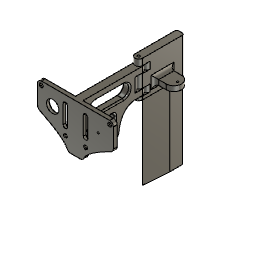
rudder (Autodesk Fusion 360 design; units mm, degrees)
Autodesk Fusion 360 part; units mm, degrees
sketch "Sketch1" plane through (0, 0, 0) normal (0, 0, 1) x (1, 0, 0)
  line L0 (0, 0) -> (60, 0)
  line L1 (60, 0) -> (60, 3)
  line L2 (0, 3) -> (0, 0)
  line L3 (30, 3) -> (30, 53) construction
  line L4 (30, 53) -> (33, 53) construction
  line L5 (30, 53) -> (27, 53) construction
  line L6 (27, 53) -> (33, 53)
  line L7 (33, 53) -> (33, 3)
  line L8 (27, 53) -> (27, 3)
  line L9 (60, 3) -> (33, 3)
  line L10 (27, 3) -> (0, 3)
  dimension "d1" = 60
  dimension "d2" = 3
  dimension "d3" = 50
  dimension "d4" = 3
  dimension "d5" = 3
  constraint horizontal L0
  constraint vertical L1
  constraint horizontal L9
  constraint vertical L2
  constraint coincident L0.start L2.end
  constraint perpendicular L3 L9
  constraint perpendicular L3 L4
  constraint perpendicular L3 L5
  constraint perpendicular L7 L9
  constraint coincident L8.end L9
  constraint perpendicular L8 L9
  constraint collinear L9 L10
  measures "d1" distance of L0.start L0.end
  measures "d2" distance of L0.start L2.start
  measures "d3" distance of L3.start L3.end
  measures "d4" distance of L3.end L4.end
  measures "d5" distance of L3.end L5.end
extrude "Extrude1" add sketch "Sketch1" along normal blind 20 makes body 1
sketch "Sketch2" plane through (33, 0, 0) normal (1, 0, 0) x (0, 1, 0)
  line L0 (3, 0) -> (53, 0)
  line L1 (53, 0) -> (53, 20)
  line L2 (53, 20) -> (3, 20)
  line L3 (3, 20) -> (3, 0)
  line L4 (53, 20) -> (53, 15.5) construction
  line L5 (53, 0) -> (53, 4.5) construction
  line L6 (53, 4.5) -> (47, 4.5)
  line L7 (47, 4.5) -> (47, 15.5)
  line L8 (47, 15.5) -> (53, 15.5)
  line L9 (53, 15.5) -> (53, 4.5)
  dimension "d8" = 4.5
  dimension "d9" = 4.5
  dimension "d10" = 6
  constraint coincident L1.end L2.start
  constraint perpendicular L2 L4
  constraint coincident L0.end L1.start
  constraint perpendicular L2 L5
  constraint horizontal L6
  constraint vertical L7
  constraint horizontal L8
  constraint vertical L9
  measures "d8" distance of L1.end L4.end
  measures "d9" distance of L0.end L5.end
  measures "d10" distance of L5.end L6.end
extrude "Extrude2" cut sketch "Sketch2" against normal blind 6 contours L1 L6 L7 L8 L9 bodies 1
fillet "Fillet2" radius 3 4 edges at (27, 53, 2.25) (27, 53, 17.75) (33, 53, 2.25) (33, 53, 17.75) on bodies 1
sketch "Sketch4" plane through (0, 0, 20) normal (0, 0, 1) x (-1, 0, 0)
  arc A0 (-33, -50) -> (-27, -50) centre (-30, -50) ccw
  line L0 (-27, -50) -> (-27, -3)
  line L1 (-27, -3) -> (0, -3)
  line L2 (0, 0) -> (-60, 0)
  line L3 (-60, -3) -> (-33, -3)
  line L4 (-33, -3) -> (-33, -50)
  circle A1 centre (-30, -50) radius 1.25
  line L5 (0, -3) -> (0, 0)
  line L6 (-60, 0) -> (-60, -3)
  dimension "d17" = 2.5
  constraint concentric A0 A1
  measures "d17" diameter of A1
extrude "Extrude3" cut sketch "Sketch4" against normal blind 20 contours A1 bodies 1
sketch "Sketch10" plane through (0, 3, 0) normal (0, 1, 0) x (-1, 0, 0)
  line L0 (-27, 0) -> (0, 0)
  line L1 (0, 0) -> (0, 20)
  line L2 (0, 20) -> (-27, 20)
  line L3 (-27, 20) -> (-27, 0)
sketch "Sketch11" plane through (0, 3, 0) normal (0, 1, 0) x (-1, 0, 0)
  line L0 (-33, 20) -> (-60, 20)
  line L1 (-60, 20) -> (-60, 0)
  line L2 (-60, 0) -> (-33, 0)
  line L3 (-33, 0) -> (-33, 20)
sketch "Sketch14" plane through (0, 0, 0) normal (1, 0, 0) x (0, 1, 0)
  line L0 (90.0644, 25) -> (120.0644, 25)
  line L1 (120.0644, 25) -> (120.0644, -65)
  line L2 (120.0644, -65) -> (90.0644, -65)
  line L3 (90.0644, 25) -> (84.0644, 25)
  line L4 (84.0644, -3.5) -> (90.0644, -3.5)
  line L5 (84.0644, 25) -> (84.0644, 20) construction
  line L6 (84.0644, -3.5) -> (84.0644, -1) construction
  line L7 (84.0644, 20) -> (84.0644, 14.5) construction
  line L8 (84.0644, 4.5) -> (90.0644, 4.4065)
  line L9 (84.0644, 14.5) -> (90.0644, 14.5)
  line L10 (84.0644, -1) -> (90.0644, -1)
  line L11 (84.0644, 20) -> (90.0645, 20)
  line L12 (84.0644, 25) -> (84.0644, 20)
  line L13 (84.0644, 14.5) -> (84.0644, 4.5)
  line L14 (84.0644, -1) -> (84.0644, -3.5)
  line L15 (90.0644, -1) -> (90.0644, 4.4065)
  line L16 (90.0644, 14.5) -> (90.0644, 20)
  line L17 (90.0644, 14.5) -> (90.0644, 20)
  line L18 (90.0644, -65) -> (90.0644, -3.5)
  line L19 (90.0644, -1) -> (90.0644, 4.4065)
  line L20 (90.0644, -3.5) -> (120.0644, -3.5)
  dimension "d43" = 30
  dimension "d44" = 90
  dimension "d45" = 6
  dimension "d46" = 28.5
  dimension "d47" = 2.5
  dimension "d48" = 5.5
  dimension "d49" = 5.5
  dimension "d50" = 6
  constraint horizontal L0
  constraint vertical L1
  constraint horizontal L2
  constraint vertical L18
  constraint horizontal L3
  constraint vertical L12
  constraint horizontal L4
  constraint vertical L15
  constraint perpendicular L4 L6
  constraint perpendicular L3 L7
  constraint horizontal L9
  constraint horizontal L10
  constraint horizontal L11
  constraint collinear L12 L13
  constraint collinear L13 L14
  constraint collinear L15 L16
  constraint collinear L17 L18
  constraint coincident L11 L16.end
  constraint coincident L10 L15.start
  constraint collinear L18 L19
  constraint coincident L1 L20.end
  constraint perpendicular L1 L20
  measures "d43" distance of L0.start L0.end
  measures "d44" distance of L0.start L2.end
  measures "d45" distance of L0.start L3.end
  measures "d46" distance of L0.start L4.end
  measures "d47" distance of L4.start L6.end
  measures "d48" distance of L6.end L8.start
  measures "d49" distance of L5.end L7.end
  measures "d50" distance of L7.end L9.end
extrude "Extrude9" add sketch "Sketch14" along normal mid plane 6 separate body contours L0 L1 L3 L4 L8 L9 L10 L11 L12 L13 L14 L15 L16 L17 L19 L20 makes body 2
extrude "Extrude10" add sketch "Sketch14" along normal mid plane 3 contours L1 L2 L18 L20 bodies 2
fillet "Fillet7" radius 3 6 edges at (-3, 84.0644, 22.5) (3, 84.0644, 22.5) (3, 84.0644, 9.5) (-3, 84.0644, 9.5) (-3, 84.0644, -2.25) (3, 84.0644, -2.25) on bodies 2
sketch "Sketch16" plane through (0, 0, 25) normal (0, 0, 1) x (-1, 0, 0)
  arc A0 (3, -87.0644) -> (-3, -87.0644) centre (0, -87.0644) ccw
  line L0 (-3, -87.0644) -> (-3, -120.0644)
  line L1 (-3, -120.0644) -> (3, -120.0644)
  line L2 (3, -120.0644) -> (3, -87.0644)
  circle A1 centre (0, -87.0644) radius 1
  dimension "d58" = 2
  constraint concentric A0 A1
  measures "d58" diameter of A1
extrude "Extrude11" cut sketch "Sketch16" against normal blind 31 contours A1 bodies 2
sketch "Sketch17" plane through (0, 0, -65) normal (0, 0, -1) x (1, 0, 0)
  line L0 (-1.5, -120.0644) -> (1.5, -120.0644)
  line L1 (1.5, -120.0644) -> (1.5, -90.0644)
  line L2 (1.5, -90.0644) -> (-1.5, -90.0644)
  line L3 (-1.5, -90.0644) -> (-1.5, -120.0644)
  line L4 (0, -90.0644) -> (0, -110.0644) construction
  line L5 (0, -110.0644) -> (1.5, -110.0644) construction
  line L6 (0, -110.0644) -> (-1.5, -110.0644) construction
  line L7 (30, 110) -> (30, 470) construction
  line L8 (0, -90.0644) -> (1.5, -110.0644)
  line L9 (0, -90.0644) -> (-1.5, -110.0644)
  dimension "d62" = 20
  constraint midpoint L2 L4.start
  constraint perpendicular L2 L4
  constraint coincident L1 L5.end
  constraint perpendicular L1 L5
  constraint coincident L3 L6.end
  constraint perpendicular L3 L6
  constraint perpendicular L6 L7
  measures "d62" distance of L4.start L4.end
extrude "Extrude12" cut sketch "Sketch17" against normal blind 61.5 contours L2 L3 L9 | L1 L2 L8 bodies 2
fillet "Fillet9" radius 1 4 edges at (0.75, 100.0644, -3.5) (1.5, 115.0644, -3.5) (-0.75, 100.0644, -3.5) (-1.5, 115.0644, -3.5) on bodies 2
fillet "Fillet10" radius 1.5 2 edges at (3, 120.0644, 10.75) (-3, 120.0644, 10.75) on bodies 2
sketch "Sketch19" plane through (3, 0, 0) normal (1, 0, 0) x (0, 1, 0)
  line L0 (118.5644, -3.5) -> (118.5644, 25)
  line L1 (118.5644, 25) -> (87.0644, 25)
  line L2 (87.0644, 25) -> (87.0644, 20)
  line L3 (87.0644, 20) -> (90.0644, 20)
  line L4 (90.0644, 20) -> (90.0644, 14.5)
  line L5 (90.0644, 14.5) -> (87.0644, 14.5)
  line L6 (87.0644, 14.5) -> (87.0644, 4.4532)
  line L7 (87.0644, 4.4532) -> (90.0644, 4.4065)
  line L8 (90.0644, 4.4065) -> (90.0644, -1)
  line L9 (90.0644, -1) -> (87.0644, -1)
  line L10 (87.0644, -1) -> (87.0644, -3.5)
  line L11 (87.0644, -3.5) -> (118.5644, -3.5)
  line L12 (87.0644, 9.4766) -> (118.5644, 10.75) construction
  line L13 (108.8144, 6.9899) -> (96.8144, 6.9899)
  line L14 (108.8144, 6.9899) -> (120, 6.9899) construction
  line L15 (108.8144, 6.9899) -> (96.8144, 6.9899)
  line L16 (96.8144, 6.9899) -> (96.8144, 2.9899)
  line L17 (96.8144, 2.9899) -> (108.8144, 2.9899)
  line L18 (108.8144, 2.9899) -> (108.8144, 6.9899)
  point P0 (102.8144, 10.1133)
  dimension "d122" = 12
  dimension "d123" = 4
  constraint midpoint L6 L12.start
  constraint midpoint L0 L12.end
  constraint horizontal L13
  constraint midpoint L12 P0
  constraint perpendicular L0 L14
  constraint horizontal L15
  constraint vertical L16
  constraint horizontal L17
  constraint vertical L18
  measures "d122" distance of L13.start L13.end
  measures "d123" distance of L13.start L17.end
extrude "Extrude14" add sketch "Sketch19" along normal blind 15 contours L13 L15 L16 L17 L18 bodies 2
fillet "Fillet14" radius 3 4 edges at (-3, 90.0644, 1.7032) (-3, 90.0644, 17.25) (3, 90.0644, 17.25) (3, 90.0644, 1.7032) on bodies 2
sketch "Sketch23" plane through (0, 0, 0) normal (0, -1, 0) x (1, 0, 0)
  line L0 (0, 20) -> (0, 0)
  line L1 (0, 0) -> (60, 0)
  line L2 (60, 0) -> (60, 20)
  line L3 (60, 20) -> (0, 20)
  line L4 (3, 17) -> (57, 17) construction
  line L5 (30, 17) -> (57, 17) construction
  line L6 (57, 17) -> (3, 17) construction
  line L7 (30, 20) -> (30, -30) construction
  circle A0 centre (3, 17) radius 1.5
  circle A1 centre (57, 17) radius 1.5
  line L8 (18, 0) -> (42, 0)
  line L9 (30, 17) -> (30, -8) construction
  line L10 (30, -8) -> (38, -8) construction
  line L11 (30, -8) -> (22, -8) construction
  circle A2 centre (38, -8) radius 1.5
  circle A3 centre (22, -8) radius 1.5
  line L12 (30, -18) -> (24, -18)
  line L13 (30, -18) -> (36, -18)
  spline S0 degree 5 poles (24, -18) (23.9428, -17.6951) (23.7865, -17.08) (23.4264, -16.1409) (22.6907, -14.8553) (21.3234, -13.1901) (19.4864, -11.4635) (17.1816, -9.6759) (14.4461, -7.8321) (11.3264, -5.9383) (7.8686, -4.0003) (4.8605, -2.4184) (2.4785, -1.2155) (0.8353, -0.4064) (0, 0) knots 0 0 0 0 0 0 0.1 0.2 0.3 0.4 0.5 0.6 0.7 0.8 0.9 1 1 1 1 1 1
  spline S1 degree 5 poles (36, -18) (36.0572, -17.6951) (36.2135, -17.08) (36.5736, -16.1409) (37.3093, -14.8553) (38.6766, -13.1901) (40.5136, -11.4635) (42.8184, -9.6759) (45.5539, -7.8321) (48.6736, -5.9383) (52.1314, -4.0003) (55.1395, -2.4184) (57.5215, -1.2155) (59.1647, -0.4064) (60, 0) knots 0 0 0 0 0 0 0.1 0.2 0.3 0.4 0.5 0.6 0.7 0.8 0.9 1 1 1 1 1 1
  line L14 (24.4672, -20.4896) -> (23.5328, -15.5104)
  line L15 (3.7531, -1.8254) -> (-3.7531, 1.8254)
  line L16 (35.5328, -20.4896) -> (36.4672, -15.5104)
  line L17 (56.2469, -1.8254) -> (63.7531, 1.8254)
  point P0 (18, 0)
  point P1 (42, 0)
  point P2 (30, -18)
  point P3 (20, -12)
  point P4 (40, -12)
  dimension "d89" = 3
  dimension "d90" = 3
  dimension "d93" = 12
  dimension "d94" = 12
  dimension "d171" = 25
  dimension "d172" = 8
  dimension "d173" = 8
  dimension "d174" = 3
  dimension "d175" = 3
  dimension "d176" = 20
  dimension "d179" = 38
  dimension "d180" = 6
  dimension "d181" = 6
  constraint midpoint L4 L5.start
  constraint midpoint L3 L7.start
  constraint perpendicular L1 L7
  constraint coincident L4.start L6.end
  constraint coincident L4.end L5.end
  constraint coincident L1 P0
  constraint coincident L1 P1
  constraint horizontal L8
  constraint coincident P0 L8.start
  constraint perpendicular L1 L9
  constraint perpendicular L9 L10
  constraint perpendicular L7 L11
  constraint coincident L10.end A2.centre
  constraint coincident L11.end A3.centre
  constraint coincident L7 P2
  constraint coincident P2 L12.start
  constraint perpendicular L7 L12
  constraint perpendicular L7 L13
  constraint coincident L0.end L1.start
  constraint midpoint L12.end L14
  constraint midpoint L0.end L15
  constraint symmetric L7 L12.end L13.end
  constraint symmetric L7 P3 P4
  constraint symmetric L7 L0.end L1.end
  constraint symmetric L7 L14.start L16.start
  constraint symmetric L7 L14.end L16.end
  constraint symmetric L7 L15.start L17.start
  constraint symmetric L7 L15.end L17.end
  measures "d89" diameter of A0
  measures "d90" diameter of A1
  measures "d93" distance of L7 P0
  measures "d94" distance of L7 P1
  measures "d171" distance of L5.start L9.end
  measures "d172" distance of L9.end L10.end
  measures "d173" distance of L9.end L11.end
  measures "d174" diameter of A2
  measures "d175" diameter of A3
  measures "d176" distance of L0.end L0.start
  measures "d179" distance of L7.start P2
  measures "d180" distance of P2 L12.end
  measures "d181" distance of P2 L13.end
extrude "Extrude17" add sketch "Sketch23" against normal blind 3 contours L0 L1 L2 L3 L8 | A0 | A1 bodies 1
extrude "Extrude18" cut sketch "Sketch23" against normal blind 3 contours A0 | A1 bodies 1
fillet "Fillet15" radius 3 2 edges at (33, 47, 10) (27, 47, 10) on bodies 1
sketch "Sketch24" plane through (0, 3, 0) normal (0, 1, 0) x (-1, 0, 0)
  circle A0 centre (-3, 17) radius 1.5
  circle A1 centre (-57, 17) radius 1.5
  line L0 (0, 20) -> (-27, 20)
  line L1 (-60, 20) -> (-60, 0)
  line L2 (0, 0) -> (0, 20)
  line L3 (-60, 0) -> (-33, 0)
  line L4 (-57, 17) -> (-48, 17) construction
  line L5 (-48, 17) -> (-48, 7) construction
  circle A2 centre (-48, 7) radius 2
  circle A3 centre (-48, 7) radius 0.75
  line L6 (-27, 20) -> (-27, 0)
  line L7 (-33, 0) -> (-33, 20)
  line L8 (-33, 20) -> (-60, 20)
  line L9 (-27, 0) -> (0, 0)
  point P0 (-30, 17)
  dimension "d101" = 9
  dimension "d102" = 10
  dimension "d103" = 4
  dimension "d109" = 18
  dimension "d116" = 1.5
  constraint coincident A1.centre L4.start
  constraint parallel L0 L4
  constraint perpendicular L4 L5
  constraint coincident L5.end A2.centre
  measures "d101" distance of A1.centre L4.end
  measures "d102" distance of L4.end L5.end
  measures "d103" diameter of A2
  measures "d109" distance of L4.end P0
  measures "d116" diameter of A3
ref_plane "WorkPlane1" through (3, 13, 17) normal (0, 1, 0) x (-1, 0, 0)
sketch "Sketch27" plane through (48, 13, 7) normal (0, 1, 0) x (1, 0, 0)
  circle A0 centre (0, 0) radius 1.5
  dimension "d115" = 3
  constraint coincident A0.centre origin
  measures "d115" diameter of A0
loft "Loft4" add profiles "Sketch24", "Sketch27" section 1 contours A2 | A3 section 2 bodies 1
extrude "Extrude21" cut sketch "Sketch24" along normal blind 12 and the other way blind 3 contours A3 bodies 1
fillet "Fillet16" radius 3 1 edges at (49.8647, 3, 7.7232) on bodies 1
sketch "Sketch28" plane through (0, 0, 6.9899) normal (0, 0, 1) x (-1, 0, 0)
  line L0 (-3, -108.8144) -> (-3, -96.8144)
  line L1 (-3, -96.8144) -> (-18, -96.8144)
  line L2 (-18, -96.8144) -> (-18, -108.8144)
  line L3 (-18, -108.8144) -> (-3, -108.8144)
  line L4 (-3, -102.8144) -> (-15, -102.8144) construction
  circle A0 centre (-15, -102.8144) radius 0.75
  dimension "d124" = 12
  dimension "d125" = 1.5
  constraint midpoint L0 L4.start
  constraint perpendicular L2 L4
  constraint coincident L4.end A0.centre
  measures "d124" distance of L4.start L4.end
  measures "d125" diameter of A0
extrude "Extrude22" cut sketch "Sketch28" against normal blind 4 contours A0 bodies 2
fillet "Fillet17" radius 6 2 edges at (18, 108.8144, 4.9899) (18, 96.8144, 4.9899) on bodies 2
fillet "Fillet18" radius 3 4 edges at (3, 102.8144, 6.9899) (3, 108.8144, 4.9899) (3, 102.8144, 2.9899) (3, 96.8144, 4.9899) on bodies 2
sketch "Sketch29" plane through (30, 3, 0) normal (0, 1, 0) x (-1, 0, 0)
  line L0 (0, -20.8667) -> (0, 0) construction
  circle A0 centre (-18, 7) radius 4.8537
  line L1 (0, 20) -> (0, -30)
  circle A1 centre (18, 7) radius 4.8537
  point P0 (0, -9.8667)
  point P1 (0, -3.8667)
  point P2 (0, -3.8667)
  point P3 (0, -9.8667)
  constraint coincident L0.end origin
  constraint vertical L0
  constraint coincident L0 P0
  constraint coincident L0 P2
  constraint coincident P2 P1
  constraint coincident P0 P3
  constraint symmetric A0 L1 A1
sketch "Sketch30" plane through (33, 0, 0) normal (1, 0, 0) x (0, 1, 0)
  line L0 (44, 15.5) -> (50, 15.5)
  line L1 (50, 15.5) -> (50, 20)
  line L2 (50, 20) -> (3, 20)
  line L3 (3, 20) -> (3, 0)
  line L4 (3, 0) -> (50, 0)
  line L5 (50, 0) -> (50, 4.5)
  line L6 (50, 4.5) -> (44, 4.5)
  line L7 (44, 4.5) -> (44, 15.5)
  line L8 (3, 20) -> (31, 20) construction
  line L9 (3, 20) -> (3, -18) construction
  line L10 (3, -18) -> (3, 0)
  line L11 (3, 0) -> (31, 0)
  line L12 (31, 0) -> (43, 0)
  line L13 (9, 0) -> (9, -18.4286) construction
  line L14 (17.5, 0) -> (17.5, -18.9835) construction
  line L15 (26, 0) -> (26, -19.5556) construction
  line L16 (6.5, -3.5) -> (6.5, -12.9286)
  arc A0 (6.5, -12.9286) -> (11.5, -12.9286) centre (9, -12.9286) ccw
  line L17 (11.5, -12.9286) -> (11.5, -3.5)
  arc A1 (11.5, -3.5) -> (6.5, -3.5) centre (9, -3.5) ccw
  line L18 (9, -1) -> (9, -15.4286) construction
  line L19 (15, -3.5) -> (15, -13.4835)
  arc A2 (15, -13.4835) -> (20, -13.4835) centre (17.5, -13.4835) ccw
  line L20 (20, -13.4835) -> (20, -3.5)
  arc A3 (20, -3.5) -> (15, -3.5) centre (17.5, -3.5) ccw
  line L21 (17.5, -1) -> (17.5, -15.9835) construction
  line L22 (23.5, -3.5) -> (23.5, -14.0556)
  arc A4 (23.5, -14.0556) -> (28.5, -14.0556) centre (26, -14.0556) ccw
  line L23 (28.5, -14.0556) -> (28.5, -3.5)
  arc A5 (28.5, -3.5) -> (23.5, -3.5) centre (26, -3.5) ccw
  line L24 (26, -1) -> (26, -16.5556) construction
  line L25 (44, 10) -> (3, 10) construction
  line L26 (13, 5) -> (35, 5)
  arc A6 (35, 5) -> (35, 15) centre (35, 10) ccw
  line L27 (35, 15) -> (13, 15)
  arc A7 (13, 15) -> (13, 5) centre (13, 10) ccw
  line L28 (8, 10) -> (40, 10) construction
  line L29 (31, 20) -> (31, -19) construction
  line L30 (3, -18) -> (31, -19)
  spline S0 degree 5 poles (31, -19) (31.0483, -18.3567) (31.1609, -17.0921) (31.3778, -15.261) (31.7645, -12.9536) (32.4223, -10.3089) (33.2722, -7.928) (34.3339, -5.8381) (35.6241, -4.062) (37.1446, -2.6021) (38.8825, -1.4409) (40.4347, -0.7344) (41.6846, -0.3222) (42.5553, -0.0988) (43, 0) knots 0 0 0 0 0 0 0.1 0.2 0.3 0.4 0.5 0.6 0.7 0.8 0.9 1 1 1 1 1 1
  point P0 (3, 20)
  point P1 (3, 0)
  point P2 (9, 0)
  point P3 (17.5, 0)
  point P4 (26, 0)
  point P5 (9, -15.4286)
  point P6 (17.5, -15.9835)
  point P7 (26, -16.5556)
  point P8 (9, -1)
  point P9 (17.5, -1)
  point P10 (26, -1)
  point P11 (8, 10)
  point P12 (40, 10)
  point P13 (35, -5)
  dimension "d140" = 28
  dimension "d141" = 38
  dimension "d143" = 6
  dimension "d144" = 8.5
  dimension "d145" = 8.5
  dimension "d146" = 3
  dimension "d147" = 3
  dimension "d148" = 3
  dimension "d149" = 1
  dimension "d150" = 1
  dimension "d151" = 1
  dimension "d152" = 5
  dimension "d153" = 5
  dimension "d154" = 5
  dimension "d155" = 5
  dimension "d156" = 4
  dimension "d157" = 10
  dimension "d187" = 39
  constraint coincident P0 L2.end
  constraint perpendicular L3 L8
  constraint perpendicular L2 L9
  constraint coincident P1 L3.end
  constraint coincident L4 L12.end
  constraint coincident L4 P2
  constraint coincident L11 P3
  constraint coincident L4 P4
  constraint coincident P2 L13.start
  constraint perpendicular L11 L13
  constraint coincident P3 L14.start
  constraint perpendicular L11 L14
  constraint coincident P4 L15.start
  constraint perpendicular L4 L15
  constraint coincident L13 P5
  constraint coincident L14 P6
  constraint coincident L15 P7
  constraint coincident L13 P8
  constraint coincident L14 P9
  constraint coincident L15 P10
  constraint tangent L16 A0
  constraint tangent A0 L17
  constraint parallel L16 L17
  constraint tangent L17 A1
  constraint tangent L16 A1
  constraint midpoint A1 P8
  constraint midpoint A0 P5
  constraint coincident P5 L18.end
  constraint coincident P8 L18.start
  constraint tangent L19 A2
  constraint tangent A2 L20
  constraint parallel L19 L20
  constraint tangent L20 A3
  constraint tangent L19 A3
  constraint midpoint A3 P9
  constraint midpoint A2 P6
  constraint coincident P6 L21.end
  constraint perpendicular L4 L21
  constraint coincident P9 L21.start
  constraint tangent L22 A4
  constraint tangent A4 L23
  constraint parallel L22 L23
  constraint tangent L23 A5
  constraint tangent L22 A5
  constraint midpoint A5 P10
  constraint midpoint A4 P7
  constraint coincident P7 L24.end
  constraint parallel L15 L24
  constraint coincident P10 L24.start
  constraint midpoint L7 L25.start
  constraint midpoint L3 L25.end
  constraint coincident L25 P11
  constraint coincident L25 P12
  constraint tangent L26 A6
  constraint tangent A6 L27
  constraint parallel L26 L27
  constraint tangent L27 A7
  constraint tangent L26 A7
  constraint midpoint A7 P11
  constraint midpoint A6 P12
  constraint coincident P12 L28.end
  constraint coincident P11 L28.start
  constraint perpendicular L2 L29
  measures "d140" distance of P0 L8.end
  measures "d141" distance of P0 L9.end
  measures "d143" distance of P1 P2
  measures "d144" distance of P2 P3
  measures "d145" distance of P3 P4
  measures "d146" distance of L13.end P5
  measures "d147" distance of L14.end P6
  measures "d148" distance of L15.end P7
  measures "d149" distance of P2 P8
  measures "d150" distance of P3 P9
  measures "d151" distance of P4 P10
  measures "d152" diameter of A0
  measures "d153" diameter of A2
  measures "d154" diameter of A4
  measures "d155" distance of L25.end P11
  measures "d156" distance of L25.start P12
  measures "d157" diameter of A6
  measures "d187" distance of L8.end L29.end
extrude "Extrude24" add sketch "Sketch30" against normal blind 6 contours L4 L10 L11 L12 L30 S0 bodies 1
extrude "Extrude25" cut sketch "Sketch30" against normal blind 6 contours L26 A6 L27 A7 bodies 1
fillet "Fillet21" radius 1 32 edges at (33, 28.5, -8.7778) (33, 26, -16.5556) (33, 23.5, -8.7778) (33, 26, -1) (33, 20, -8.4918) (33, 17.5, -15.9835) (33, 15, -8.4918) (33, 17.5, -1) (33, 11.5, -8.2143) (33, 9, -15.4286) (33, 6.5, -8.2143) (33, 9, -1) (33, 24, 15) (33, 40, 10) (33, 24, 5) (33, 8, 10) (27, 23.5, -8.7778) (27, 26, -16.5556) (27, 28.5, -8.7778) (27, 26, -1) (27, 20, -8.4918) (27, 17.5, -1) (27, 15, -8.4918) (27, 17.5, -15.9835) (27, 11.5, -8.2143) (27, 9, -1) (27, 6.5, -8.2143) (27, 9, -15.4286) (27, 24, 15) (27, 8, 10) (27, 24, 5) (27, 40, 10) on bodies 1
extrude "Extrude27" cut sketch "Sketch23" against normal blind 3 contours A2 | A3 bodies 1
extrude "Extrude28" add sketch "Sketch23" against normal blind 3 contours L1 L8 L12 L13 S0 S1 bodies 1
fillet "Fillet23" radius 3 7 edges at (30, 31, -19) (36, 1.5, -18) (24, 1.5, -18) (60, 1.5, 0) (60, 1.5, 20) (0, 1.5, 20) (0, 1.5, 0) on bodies 1
chamfer "Chamfer2" distance 1 distance2 2 4 edges at (55.6015, 3, 16.4576) (1.6015, 3, 16.4576) (20.6015, 3, -8.5424) (36.6015, 3, -8.5424) measured on face at (37.737, 3, 6.7242) measured on face at (13.4946, 3, 10.4554) measured on face at (13.4946, 3, 10.4554) measured on face at (37.737, 3, 6.7242) on bodies 1
extrude "Extrude30" cut sketch "Sketch29" against normal blind 3 contours A1 bodies 1
fillet "Fillet25" radius 1 1 edges at (16.5253, 3, 8.7552) on bodies 1
sketch "Sketch33" plane through (0, 3, 0) normal (0, 1, 0) x (-1, 0, 0)
  circle A0 centre (-57, 17) radius 2.5
  circle A1 centre (-48, 7) radius 4.8537
  arc A2 (-57, 20) -> (-60, 17) centre (-57, 17) ccw
  line L0 (-60, 17) -> (-60, 1.8686)
  spline S0 degree 3 poles (-58.3335, -0.8187) (-58.6834, -0.645) (-58.9961, -0.4047) (-59.4924, 0.1603) (-59.6799, 0.4726) (-59.9347, 1.1489) (-60, 1.5073) (-60, 1.8686) knots 0 0 0 0 0.117193 0.117193 0.225599 0.225599 0.334005 0.334005 0.334005 0.334005
  spline S1 degree 5 poles (-58.3335, -0.8187) (-57.8493, -1.059) (-56.5651, -1.701) (-54.5337, -2.7379) (-51.8518, -4.157) (-48.6736, -5.9383) (-45.5539, -7.8321) (-42.8184, -9.6759) (-40.5136, -11.4635) (-38.7143, -13.1546) (-37.6391, -14.4539) (-37.0281, -15.3952) (-36.7062, -16.0014) (-36.5712, -16.2859) knots -0.959561 -0.959561 -0.959561 -0.959561 -0.959561 -0.959561 -0.9 -0.8 -0.7 -0.6 -0.5 -0.4 -0.3 -0.2 -0.110267 -0.110267 -0.110267 -0.110267 -0.110267 -0.110267
  spline S2 degree 3 poles (-33.8608, -18) (-34.2514, -18) (-34.6383, -17.9237) (-35.3423, -17.6348) (-35.6558, -17.4321) (-36.1933, -16.9227) (-36.4125, -16.6204) (-36.5712, -16.2859) knots 0 0 0 0 0.117193 0.117193 0.228267 0.228267 0.339341 0.339341 0.339341 0.339341
  line L1 (-33.8608, -18) -> (-33, -18)
  line L2 (-33, -18) -> (-33, 20)
  line L3 (-33, 20) -> (-57, 20)
  circle A3 centre (-38, -8) radius 2.5
  line L4 (-39.75, 13.25) -> (-39.75, -1.25)
  arc A4 (-39.75, -1.25) -> (-36.25, -1.25) centre (-38, -1.25) ccw
  line L5 (-36.25, -1.25) -> (-36.25, 13.25)
  arc A5 (-36.25, 13.25) -> (-39.75, 13.25) centre (-38, 13.25) ccw
  line L6 (-38, 15) -> (-38, -3) construction
  line L7 (-30, 20) -> (-30, -30)
  line L8 (-30, 17) -> (-30, -8)
  line L9 (-23.75, -1.25) -> (-23.75, 13.25)
  line L10 (-20.25, 13.25) -> (-20.25, -1.25)
  arc A6 (-20.25, 13.25) -> (-23.75, 13.25) centre (-22, 13.25) ccw
  arc A7 (-23.75, -1.25) -> (-20.25, -1.25) centre (-22, -1.25) ccw
  dimension "d195" = 3.5
  constraint tangent L4 A4
  constraint tangent A4 L5
  constraint parallel L4 L5
  constraint tangent L5 A5
  constraint tangent L4 A5
  constraint midpoint A5 L6.start
  constraint midpoint A4 L6.end
  constraint vertical L6
  constraint symmetric L4.start L8 L10.start
  constraint symmetric L4.end L8 L10.end
  constraint symmetric A4.end L8 L9.start
  constraint symmetric L5.end L8 L9.end
  constraint symmetric A4 L8 A7
  constraint symmetric A5 L8 A6
  measures "d195" diameter of A4
extrude "Extrude31" cut sketch "Sketch33" against normal blind 3 contours L4 A4 L5 A5 | L9 L10 A6 A7 bodies 1
fillet "Fillet26" radius 1 8 edges at (36.25, 3, 6) (38, 3, -3) (39.75, 3, 6) (38, 3, 15) (23.75, 3, 6) (22, 3, 15) (20.25, 3, 6) (22, 3, -3) on bodies 1
move_body "Move1" bodies 2 to x (1, 0, 0) y (0, 1, 0) z (0, 0, 1) at (30, -37, 0.5)
